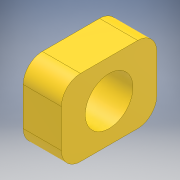
# Autodesk Inventor part: Podkladka_2mm
Saved by Autodesk Inventor 2017 (Build 210142000, 142)
## iProperties
Created: 2016-11-14
Part Number: Podkladka_2mm
Material: Generic
Document SubType Name: Modeling
Designer: Shichi
Density: 1 g/cm^3
Appearance: Glossy - Gold
Author: Shichi
Autodesk Inventor part; units mm, degrees
ref_plane "YZ Plane" through (0, 0, 0) normal (1, 0, 0) x (0, 1, 0)
ref_plane "XZ Plane" through (0, 0, 0) normal (0, 1, 0) x (-1, 0, 0)
ref_plane "XY Plane" through (0, 0, 0) normal (0, 0, 1) x (1, 0, 0)
sketch "Sketch1" plane through (0, 0, 0) normal (1, 0, 0) x (0, 1, 0)
  line L0 (1.5, 2) -> (-1.5, 2)
  line L1 (-2.5, 1) -> (-2.5, -1)
  line L2 (-1.5, -2) -> (1.5, -2)
  line L3 (2.5, -1) -> (2.5, 1)
  circle A0 centre (0, 0) radius 1.25
  arc A1 (2.5, 1) -> (1.5, 2) centre (1.5, 1) ccw
  arc A2 (1.5, -2) -> (2.5, -1) centre (1.5, -1) ccw
  arc A3 (-1.5, 2) -> (-2.5, 1) centre (-1.5, 1) ccw
  arc A4 (-2.5, -1) -> (-1.5, -2) centre (-1.5, -1) ccw
  point P0 (2.5, 2)
  point P1 (-2.5, 2)
  point P2 (2.5, -2)
  point P3 (2.5, 0)
  point P4 (0, 2)
  dimension "d0" = 4
  dimension "d1" = 5
  dimension "d2" = 2.5
  dimension "d3" = 1
  constraints: 8 end point, 8 point on circle, 8 tangent, 6 point on line, 5 centre point, 3 equal radius, 2 midpoint, 2 parallel, 1 coincident, 1 horizontal, 1 horizontal alignment, 1 perpendicular, 1 vertical alignment
  measures "d0" distance of point (2.5, -2) point (2.5, 2)
  measures "d1" distance of point (2.5, 2) point (-2.5, 2)
  measures "d2" diameter of A0
  measures "d3" radius of A1
extrude "Extrusion1" add sketch "Sketch1" along normal blind 2
body "Solid1"
